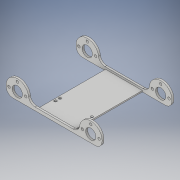
# Autodesk Inventor part: Servo Plate V3
Saved by Autodesk Inventor 2019 (Build 230136000, 136)
## iProperties
Created: 2018-11-14
Part Number: Servo Plate V3
Material: Generic
Document SubType Name: Modeling
Designer: Ashley
Density: 1 g/cm^3
Appearance: Default
Author: Ashley
Autodesk Inventor part; units mm, degrees
ref_plane "YZ Plane" through (0, 0, 0) normal (1, 0, 0) x (0, 1, 0)
ref_plane "XZ Plane" through (0, 0, 0) normal (0, 1, 0) x (-1, 0, 0)
ref_plane "XY Plane" through (0, 0, 0) normal (0, 0, 1) x (1, 0, 0)
sketch "Main Body Sketch" plane through (0, 0, 0) normal (0, 1, 0) x (-1, 0, 0)
  line L0 (-28.5, -55.75) -> (28.5, -55.75)
  line L1 (28.5, -55.75) -> (28.5, 55.75)
  line L2 (28.5, 55.75) -> (-28.5, 55.75)
  line L3 (-28.5, 55.75) -> (-28.5, -55.75)
  line L4 (-28.5, -55.75) -> (28.5, 55.75) construction
  line L5 (28.5, -55.75) -> (-28.5, 55.75) construction
  line L6 (0, 72.0987) -> (0, -84.1537) construction
  circle A0 centre (-24.75, 28.75) radius 2
  circle A1 centre (24.75, 28.75) radius 2
  circle A2 centre (24.75, 21.75) radius 2
  circle A3 centre (-24.75, 21.75) radius 2
  point P0 (0, 0)
  dimension "d0" = 57
  dimension "d1" = 111.5
  dimension "d2" = 4
  dimension "d3" = 24.75
  dimension "d4" = 27
  dimension "d7" = 7
  constraints: 14 end point, 4 centre point, 2 midpoint, 2 parallel, 2 symmetric about line, 1 horizontal, 1 perpendicular, 1 vertical, 2 other
  measures "d0" distance between parallel lines of L3 L1
  measures "d1" distance between parallel lines of L0 L2
  measures "d2" diameter of A0
  measures "d3" distance from line of L6 A0.centre
  measures "d4" distance from line of L2 A0.centre
  measures "d7" distance of A1.centre A2.centre
extrude "Main Body Extrusion" add sketch "Main Body Sketch" along normal blind 2
sketch "Mounting Circles" plane through (-28.5, 0, 55.75) normal (0, 0, 1) x (1, 0, 0)
  circle A0 centre (-28.5, 12) radius 8
  arc A1 (-12.457, 5.0091) -> (-41.2377, 0) centre (-28.5, 12) ccw
  line L0 (-12.457, 5.0091) -> (0, 5.0091)
  line L1 (28.5, -10.7409) -> (28.5, 31.3182) construction
  circle A2 centre (-28.5, 25) radius 2
  circle A3 centre (-41.5, 12) radius 2
  circle A4 centre (-15.5, 12) radius 2
  circle A5 centre (85.5, 12) radius 8
  arc A6 (98.2377, 0) -> (69.457, 5.0091) centre (85.5, 12) ccw
  line L2 (69.457, 5.0091) -> (57, 5.0091)
  line L3 (57, 0) -> (57, 2) construction
  circle A7 centre (85.5, 25) radius 2
  circle A8 centre (98.5, 12) radius 2
  circle A9 centre (72.5, 12) radius 2
  line L4 (0, 5.0091) -> (57, 5.0091)
  line L5 (0, 0) -> (0, 2) construction
  line L6 (57, 0) -> (0, 0) construction
  line L7 (-41.2377, 0) -> (98.2377, 0)
  point P0 (28.5, 0)
  dimension "d10" = 57
  dimension "d11" = 16
  dimension "d13" = 35
  dimension "d19" = 4
  dimension "d20" = 4
  dimension "d21" = 4
  dimension "d22" = 13
  dimension "d23" = 13
  dimension "d24" = 13
  constraints: 12 end point, 10 centre point, 10 symmetric about line, 4 point on circle, 2 coincident, 1 collinear, 1 horizontal, 1 vertical, 5 other
  measures "d10" horizontal distance of point (28.5, 0) A0.centre
  measures "d11" diameter of A0
  measures "d13" diameter of A1
  measures "d19" diameter of A4
  measures "d20" diameter of A2
  measures "d21" diameter of A3
  measures "d22" distance of A4.centre A0.centre
  measures "d23" distance of A0.centre A2.centre
  measures "d24" distance of A0.centre A3.centre
extrude "Side Attatchments" add sketch "Mounting Circles" against normal blind 3
fillet "Fillet5" radius 10 2 edges at (-40.957, 5.0091, 54.25) (40.957, 5.0091, 54.25)
fillet "Fillet6" radius 10 2 edges at (-69.7377, 0, 54.25) (69.7377, 0, 54.25)
mirror "Mirror1" about plane through (0, 0, 0) normal (0, 0, 1) of "Side Attatchments"
fillet "Fillet7" radius 10 4 edges at (-40.957, 5.0091, -54.25) (40.957, 5.0091, -54.25) (-69.7377, 0, -54.25) (69.7377, 0, -54.25)
ref_plane "Work Plane1" through (0, 0, 0) normal (0, 0, 1) x (1, 0, 0)
body "Solid2"
